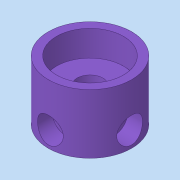
# Autodesk Inventor part: SpoolCarrageMagnetMountREV2
Saved by Autodesk Inventor 2017.3 (Build 213256000, 256)
## iProperties
Created: 2019-01-08
Part Number: SpoolCarrageMagnetMountREV2
Material: ABS Plastic
Document SubType Name: Modeling
Designer: Derek Wider
Density: 1.06 g/cm^3
Appearance: Violet
Author: Derek Wider
Autodesk Inventor part; units mm, degrees
ref_plane "XZ Plane" through (0, 0, 0) normal (0, 1, 0) x (-1, 0, 0)
ref_plane "XY Plane" through (0, 0, 0) normal (0, 0, 1) x (1, 0, 0)
sketch "Sketch1" plane through (0, 0, 0) normal (0, 1, 0) x (-1, 0, 0)
  circle A0 centre (0, 0) radius 4.2926
  circle A1 centre (0, 0) radius 5.334
  dimension "d0" = 8.5852
  dimension "d1" = 10.668
  constraints: 2 centre point, 2 coincident
  measures "d0" diameter of A0
  measures "d1" diameter of A1
extrude "Extrusion1" add sketch "Sketch1" along normal blind 3.302
sketch "Sketch2" plane through (0, 0, 0) normal (0, -1, 0) x (1, 0, 0)
  circle A0 centre (0, 0) radius 5.334 projected
  circle A1 centre (0, 0) radius 1.651
  dimension "d4" = 3.302
  constraints: 1 centre point, 1 coincident
  measures "d4" diameter of A1
extrude "Extrusion2" add sketch "Sketch2" along normal blind 4.318
ref_plane "Work Plane1" through (-5.334, 0, 0) normal (1, 0, 0) x (0, 1, 0)
sketch "Sketch3" plane through (-5.334, 0, 0) normal (1, 0, 0) x (0, 1, 0)
  circle A0 centre (-2.286, 0) radius 1.651
  line L0 (-4.318, 5.334) -> (-4.318, -5.334) projected
  point P0 (0, 0)
  dimension "d7" = 3.302
  dimension "d8" = 2.032
  constraints: 1 centre point
  measures "d7" diameter of A0
  measures "d8" distance from line of L0 A0.centre
extrude "Extrusion3" cut sketch "Sketch3" along normal blind 2.159
pattern_circular "Circular Pattern1" count 4 over 360 about axis through (0, 0, 0) along (0, 1, 0) of "Extrusion3"
body "Solid1"
